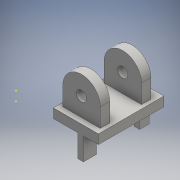
# Autodesk Inventor part: sail_hold_1
Saved by Autodesk Inventor 2016 (Build 200138000, 138)
## iProperties
Created: 2015-09-21
Part Number: sail_hold_1
Material: Generic
Document SubType Name: Modeling
Designer: Qiuyang
Density: 1 g/cm^3
Appearance: Default
Author: Qiuyang
Autodesk Inventor part; units mm, degrees
ref_plane "YZ Plane" through (0, 0, 0) normal (1, 0, 0) x (0, 1, 0)
ref_plane "XZ Plane" through (0, 0, 0) normal (0, 1, 0) x (-1, 0, 0)
ref_plane "XY Plane" through (0, 0, 0) normal (0, 0, 1) x (1, 0, 0)
sketch "Sketch1" plane through (0, 0, 0) normal (0, 0, 1) x (1, 0, 0)
  line L0 (0, 0) -> (60, 0)
  line L1 (60, 0) -> (60, 37)
  line L2 (60, 37) -> (0, 37)
  line L3 (0, 37) -> (0, 0)
  dimension "d0" = 60
  dimension "d1" = 37
  constraints: 8 end point, 2 parallel, 1 horizontal, 1 perpendicular
  measures "d0" distance of L2.end L1.end
  measures "d1" distance of L1.end L0.end
extrude "Extrusion1" add sketch "Sketch1" along normal blind 5
sketch "Sketch2" plane through (0, 0, 5) normal (0, 0, 1) x (1, 0, 0)
  line L0 (20, 27) -> (40, 27)
  line L1 (40, 27) -> (40, 32)
  line L2 (40, 32) -> (20, 32)
  line L3 (20, 32) -> (20, 27)
  line L4 (20, 10) -> (40, 10)
  line L5 (40, 10) -> (40, 5)
  line L6 (40, 5) -> (20, 5)
  line L7 (20, 5) -> (20, 10)
  point P0 (0, 0)
  dimension "d6" = 20
  dimension "d7" = 5
  dimension "d8" = 20
  dimension "d9" = 5
  constraints: 16 end point, 4 parallel, 2 horizontal, 2 perpendicular
  measures "d6" distance of L2.end L1.end
  measures "d7" distance of L1.end L0.end
  measures "d8" distance of L5.end L6.end
  measures "d9" distance of L4.end L5.end
extrude "Extrusion2" add sketch "Sketch2" along normal blind 20
sketch "Sketch3" plane through (20, 32, 5) normal (0, 1, 0) x (1, 0, 0)
  circle A0 centre (10, -10) radius 2.7
  point P0 (-20, 5)
  dimension "d12" = 5.4
  constraints: 1 centre point
  measures "d12" diameter of A0
extrude "Extrusion3" cut sketch "Sketch3" against normal blind 20
sketch "Sketch4" plane through (20, 10, 5) normal (0, 1, 0) x (1, 0, 0)
  circle A0 centre (10, -10) radius 2.7
  point P0 (-20, 5)
  dimension "d15" = 5.4
  constraints: 1 centre point
  measures "d15" diameter of A0
extrude "Extrusion4" cut sketch "Sketch4" against normal blind 20
fillet "Fillet1" radius 10 1 edges at (40, 29.5, 25)
fillet "Fillet2" radius 10 1 edges at (20, 29.5, 25)
fillet "Fillet3" radius 10 1 edges at (40, 7.5, 25)
fillet "Fillet4" radius 10 1 edges at (20, 7.5, 25)
sketch "Sketch5" plane through (0, 0, 5) normal (0, 0, 1) x (1, 0, 0)
  circle A0 centre (10, 10) radius 2.5
  circle A1 centre (50, 10) radius 2.5
  circle A2 centre (10, 27) radius 2.5
  circle A3 centre (50, 27) radius 2.5
  point P0 (0, 0)
  dimension "d22" = 5
  dimension "d23" = 5
  dimension "d24" = 5
  dimension "d25" = 5
  constraints: 4 centre point
  measures "d22" diameter of A0
  measures "d23" diameter of A1
  measures "d24" diameter of A2
  measures "d25" diameter of A3
extrude "Extrusion5" cut sketch "Sketch5" against normal blind 20
fillet "Fillet5" radius 10 1 edges at (0, 37, 2.5)
fillet "Fillet6" radius 10 1 edges at (60, 37, 2.5)
fillet "Fillet7" radius 10 1 edges at (60, 0, 2.5)
fillet "Fillet8" radius 10 1 edges at (0, 0, 2.5)
sketch "Sketch6" plane through (0, 0, 0) normal (0, 0, -1) x (-1, 0, 0)
  point P0 (0, 0)
sketch "Sketch7" plane through (0, 0, 5) normal (0, 0, 1) x (1, 0, 0)
  line L0 (10, 0) -> (50, 0) projected
  line L1 (50, 37) -> (10, 37) projected
  line L2 (18, 0) -> (42, 0)
  line L3 (42, 0) -> (42, 37)
  line L4 (42, 37) -> (18, 37)
  line L5 (18, 37) -> (18, 0)
  line L6 (18, 0) -> (0, 0)
  line L7 (0, 0) -> (0, 37)
  line L8 (0, 37) -> (18, 37)
  line L9 (18, 37) -> (18, 0)
  line L10 (42, 0) -> (60, 0)
  line L11 (60, 0) -> (60, 37)
  line L12 (60, 37) -> (42, 37)
  line L13 (42, 37) -> (42, 0)
  dimension "d32" = 24
  constraints: 24 end point, 6 parallel, 4 point on line, 3 horizontal, 3 perpendicular
  measures "d32" distance of L4.end L3.end
extrude "Extrusion6" cut sketch "Sketch7" against normal blind 10 contours L6 L7 L8 L1 L5 L0 | L3 L1 L12 L11 L10 L0
sketch "Sketch8" plane through (0, 0, 0) normal (0, 0, -1) x (-1, 0, 0)
  point P0 (0, 0)
sketch "Sketch9" plane through (0, 0, 0) normal (0, 0, -1) x (-1, 0, 0)
  line L0 (-18, 0) -> (-42, 0) projected
  line L1 (-34, 0) -> (-31, 0)
  line L2 (-31, 0) -> (-31, 9)
  line L3 (-31, 9) -> (-34, 9)
  line L4 (-34, 9) -> (-34, 0)
  line L5 (-18, 0) -> (-18, 37) projected
  point P0 (0, 0)
  point P1 (-23, 0)
  point P2 (-37, 0)
  point P3 (-18, 5)
  point P4 (-18, 32)
  dimension "d36" = 3
  dimension "d37" = 9
  dimension "d38" = 16
  constraints: 8 end point, 2 parallel, 1 horizontal, 1 perpendicular, 1 point on line
  measures "d36" distance of L3.end L2.end
  measures "d37" distance of L2.end L1.end
  measures "d38" distance between parallel lines of L5 L4
sketch "Sketch10" plane through (0, 0, 0) normal (0, 0, -1) x (-1, 0, 0)
  line L0 (-42, 37) -> (-18, 37) projected
  line L1 (-34, 37) -> (-31, 37)
  line L2 (-31, 37) -> (-31, 32)
  line L3 (-31, 32) -> (-34, 32)
  line L4 (-34, 32) -> (-34, 37)
  line L5 (-18, 0) -> (-18, 37) projected
  point P0 (0, 0)
  dimension "d39" = 3
  dimension "d40" = 5
  dimension "d41" = 16
  constraints: 8 end point, 2 parallel, 1 horizontal, 1 perpendicular, 1 point on line
  measures "d39" distance of L2.end L3.end
  measures "d40" distance of L1.end L2.end
  measures "d41" distance between parallel lines of L5 L4
sketch "Sketch11" plane through (0, 0, 0) normal (0, 0, -1) x (-1, 0, 0)
  point P0 (0, 0)
sketch "Sketch12" plane through (0, 0, 5) normal (0, 0, 1) x (1, 0, 0)
  point P0 (0, 0)
sketch "Sketch13" plane through (0, 0, 5) normal (0, 0, 1) x (1, 0, 0)
  point P0 (0, 0)
sketch "Sketch14" plane through (0, 0, 5) normal (0, 0, 1) x (1, 0, 0)
  line L0 (42, 0) -> (42, 37) projected
  line L1 (18, 0) -> (18, 37) projected
  line L2 (42, 0) -> (18, 0)
  line L3 (18, 0) -> (18, 2)
  line L4 (18, 2) -> (42, 2)
  line L5 (42, 2) -> (42, 0)
  point P0 (0, 0)
  dimension "d42" = 2
  constraints: 8 end point, 2 parallel, 1 horizontal, 1 perpendicular, 1 point on line
  measures "d42" distance of L2.end L3.end
extrude "Extrusion7" add sketch "Sketch10" along normal blind 12
extrude "Extrusion8" add sketch "Sketch9" along normal blind 12
extrude "Extrusion9" cut sketch "Sketch14" against normal blind 22
body "Solid1"
